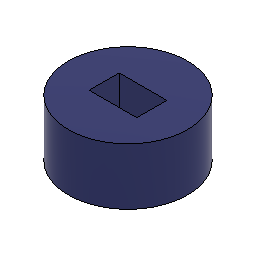
PDB tool_2023.04.26 (Autodesk Fusion 360 design; units mm, degrees)
Autodesk Fusion 360 part; units mm, degrees
sketch "Sketch1" plane through (0, 0, 0) normal (0, 1, 0) x (1, 0, 0)
  circle A0 centre (0, 0) radius 10.5
  line L0 (4.2, -2.65) -> (-4.2, -2.65)
  line L1 (-4.2, -2.65) -> (-4.2, 2.65)
  line L2 (-4.2, 2.65) -> (4.2, 2.65)
  line L3 (4.2, 2.65) -> (4.2, -2.65)
  line L4 (4.2, -2.65) -> (-4.2, 2.65) construction
  line L5 (-4.2, -2.65) -> (4.2, 2.65) construction
  dimension "d1" = 21
  dimension "d2" = 8.4
  dimension "d3" = 5.3
  constraint coincident A0.centre origin
  constraint horizontal L0
  constraint perpendicular L0 L1
  constraint parallel L0 L2
  constraint parallel L1 L3
  constraint coincident L4 A0.centre
  constraint coincident L5 A0.centre
  measures "d1" diameter of A0
  measures "d2" distance of L1.end L2.end
  measures "d3" distance of L0.end L1.end
extrude "Extrude1" add sketch "Sketch1" along normal blind 10
